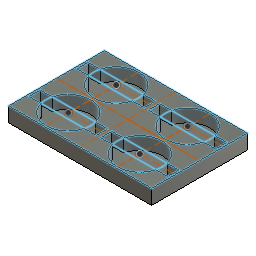
4x35mmMattek_lowspeedcentrifuge_Holder (Autodesk Fusion 360 design; units mm, degrees)
Autodesk Fusion 360 part; units mm, degrees
sketch "Sketch1" plane through (0, 0, 0) normal (0, 1, 0) x (1, 0, 0)
  line L0 (25, -25) -> (152.63, -25)
  line L1 (152.63, -25) -> (152.63, -110.47)
  line L2 (152.63, -110.47) -> (25, -110.47)
  line L3 (25, -110.47) -> (25, -25)
  line L4 (25, -67.735) -> (152.63, -67.735) construction
  line L5 (88.815, -25) -> (88.815, -110.47) construction
  line L6 (88.815, -67.735) -> (25, -67.735) construction
  line L7 (56.9075, -67.735) -> (56.9075, -25) construction
  line L8 (56.9075, -67.735) -> (56.9075, -46.3675) construction
  line L9 (88.815, -67.735) -> (152.63, -67.735) construction
  line L10 (88.815, -67.735) -> (120.7225, -67.735) construction
  line L11 (120.7225, -67.735) -> (120.7225, -25) construction
  line L12 (120.7225, -67.735) -> (120.7225, -46.3675) construction
  circle A0 centre (56.9075, -46.3675) radius 20
  circle A1 centre (120.7225, -46.3675) radius 20
  line L13 (56.9075, -67.735) -> (56.9075, -110.47) construction
  line L14 (56.9075, -67.735) -> (56.9075, -89.1025) construction
  circle A2 centre (56.9075, -89.1025) radius 20
  line L15 (120.7225, -67.735) -> (120.7225, -110.47) construction
  line L16 (120.7225, -110.47) -> (120.7225, -89.1025) construction
  circle A3 centre (120.7225, -89.1025) radius 20
  line L17 (120.7225, -46.3675) -> (150.7225, -46.3675) construction
  line L18 (150.7225, -46.3675) -> (150.7225, -41.3675) construction
  line L19 (150.7225, -41.3675) -> (90.7225, -41.3675)
  line L20 (90.7225, -41.3675) -> (90.7225, -51.3675)
  line L21 (90.7225, -51.3675) -> (150.7225, -51.3675)
  line L22 (150.7225, -51.3675) -> (150.7225, -41.3675)
  line L23 (56.9075, -46.3675) -> (86.9075, -46.3675) construction
  line L24 (86.9075, -46.3675) -> (86.9075, -41.3675) construction
  line L25 (86.9075, -41.3675) -> (26.9075, -41.3675)
  line L26 (26.9075, -41.3675) -> (26.9075, -51.3675)
  line L27 (26.9075, -51.3675) -> (86.9075, -51.3675)
  line L28 (86.9075, -51.3675) -> (86.9075, -41.3675)
  line L29 (56.9075, -89.1025) -> (86.9075, -89.1025) construction
  line L30 (86.9075, -89.1025) -> (86.9075, -84.1025) construction
  line L31 (86.9075, -84.1025) -> (26.9075, -84.1025)
  line L32 (26.9075, -84.1025) -> (26.9075, -94.1025)
  line L33 (26.9075, -94.1025) -> (86.9075, -94.1025)
  line L34 (86.9075, -94.1025) -> (86.9075, -84.1025)
  line L35 (120.7225, -89.1025) -> (150.7225, -89.1025) construction
  line L36 (150.7225, -89.1025) -> (150.7225, -84.1025) construction
  line L37 (150.7225, -84.1025) -> (90.7225, -84.1025)
  line L38 (90.7225, -84.1025) -> (90.7225, -94.1025)
  line L39 (90.7225, -94.1025) -> (150.7225, -94.1025)
  line L40 (150.7225, -94.1025) -> (150.7225, -84.1025)
  dimension "d1" = 127.63
  dimension "d2" = 85.47
  dimension "d3" = 40
  dimension "d4" = 40
  dimension "d5" = 40
  dimension "d6" = 40
  dimension "d7" = 30
  dimension "d8" = 5
  dimension "d9" = 60
  dimension "d10" = 10
  dimension "d11" = 30
  dimension "d12" = 5
  dimension "d13" = 60
  dimension "d14" = 10
  dimension "d15" = 30
  dimension "d16" = 5
  dimension "d17" = 60
  dimension "d18" = 10
  dimension "d19" = 30
  dimension "d20" = 5
  dimension "d21" = 60
  dimension "d22" = 10
  constraint horizontal L0
  constraint vertical L1
  constraint horizontal L2
  constraint vertical L3
  constraint midpoint L3 L4.start
  constraint midpoint L1 L4.end
  constraint midpoint L0 L5.start
  constraint midpoint L2 L5.end
  constraint midpoint L4 L6.start
  constraint midpoint L6 L7.start
  constraint coincident L0 L7.end
  constraint perpendicular L0 L7
  constraint midpoint L7 L8.end
  constraint midpoint L9 L10.end
  constraint coincident L0 L11.end
  constraint perpendicular L0 L11
  constraint midpoint L11 L12.end
  constraint coincident L8.end A0.centre
  constraint coincident L12.end A1.centre
  constraint coincident L2 L13.end
  constraint perpendicular L2 L13
  constraint midpoint L13 L14.end
  constraint coincident L14.end A2.centre
  constraint coincident L2 L15.end
  constraint perpendicular L2 L15
  constraint midpoint L15 L16.end
  constraint coincident L16.end A3.centre
  constraint horizontal L17
  constraint perpendicular L17 L18
  constraint horizontal L19
  constraint vertical L20
  constraint horizontal L21
  constraint vertical L22
  constraint horizontal L23
  constraint perpendicular L23 L24
  constraint horizontal L25
  constraint vertical L26
  constraint horizontal L27
  constraint vertical L28
  constraint perpendicular L13 L29
  constraint perpendicular L29 L30
  constraint horizontal L31
  constraint vertical L32
  constraint horizontal L33
  constraint vertical L34
  constraint perpendicular L15 L35
  constraint perpendicular L35 L36
  constraint horizontal L37
  constraint vertical L38
  constraint horizontal L39
  constraint vertical L40
  measures "d1" distance of L0.start L0.end
  measures "d2" distance of L0.start L2.end
  measures "d3" diameter of A0
  measures "d4" diameter of A1
  measures "d5" diameter of A2
  measures "d6" diameter of A3
  measures "d7" distance of L12.end L17.end
  measures "d8" distance of L17.end L18.end
  measures "d9" distance of L18.end L19.end
  measures "d10" distance of L18.end L21.end
  measures "d11" distance of L8.end L23.end
  measures "d12" distance of L23.end L24.end
  measures "d13" distance of L24.end L25.end
  measures "d14" distance of L24.end L27.end
  measures "d15" distance of L14.end L29.end
  measures "d16" distance of L29.end L30.end
  measures "d17" distance of L30.end L31.end
  measures "d18" distance of L30.end L33.end
  measures "d19" distance of L16.end L35.end
  measures "d20" distance of L35.end L36.end
  measures "d21" distance of L36.end L37.end
  measures "d22" distance of L36.end L39.end
extrude "Extrude1" add sketch "Sketch1" against normal blind 20.19 contours L0 L1 L2 L3 | A0 L25 L27 | A0 L25 L27 L28 | A0 L25 | A0 L27 | A0 L25 L26 L27 | A1 L19 L21 | A1 L19 L21 L22 | A1 L19 | A1 L21 | A1 L19 L20 L21 | A2 L31 L33 | A2 L31 L33 L34 | A2 L31 | A2 L33 | A2 L31 L32 L33 | A3 L37 L39 | A3 L37 L39 L40 | A3 L37 | A3 L39 | A3 L37 L38 L39
extrude "Extrude2" cut sketch "Sketch1" against normal blind 11.43 contours A0 L25 L27 | A0 L25 L27 L28 | A0 L25 | A0 L27 | A0 L25 L26 L27 | A1 L19 L21 | A1 L19 L21 L22 | A1 L19 | A1 L21 | A1 L19 L20 L21 | A2 L31 L33 | A2 L31 L33 L34 | A2 L31 | A2 L33 | A2 L31 L32 L33 | A3 L37 L39 | A3 L37 L39 L40 | A3 L37 | A3 L39
extrude "Extrude3" cut sketch "Sketch1" against normal blind 11.43 contours A3 L37 L38 L39
extrude "Extrude4" cut 1 faces at (67.5433, -20.19, 53.49) along direction (0, 1, 0) blind 7
